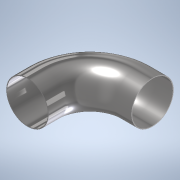
# Autodesk Inventor part: Kolano 90° ø101,6x2 R110
Saved by Autodesk Inventor 2020 (Build 240168000, 168)
## iProperties
RuleStatus: InUse
Created: 2021-10-14
Part Number: Kolano 90° ø101,6x2 R110
Material: 304L
Description: Kolano 90° ø101,6x2 R110
Document SubType Name: Modelowanie
Designer: inż. R.Jargiło
Density: 8 g/cm^3
Sheet Metal Rule: 1,5
Sheet Metal Width: 0,000 mm
Sheet Metal Length: 0,000 mm
Sheet Metal Area: 0,000 mm^2
Appearance: Częściowo polerowany(1)
Mass: 58.943 g
Surface Area: 91.7698 cm^2
Volume: 7.36788 cm^3
Project: 0479
Author: inż. R.Jargiło
Autodesk Inventor part; units mm, degrees
ref_plane "YZ Plane" through (0, 0, 0) normal (1, 0, 0) x (0, 1, 0)
ref_plane "XZ Plane" through (0, 0, 0) normal (0, 1, 0) x (-1, 0, 0)
sketch "Szkic6" plane through (0, 0, 0) normal (0, 0, 1) x (1, 0, 0)
  line L0 (-29.6067, 0) -> (35.2678, 0) construction
  line L1 (0, 42.3419) -> (0, -58.3726) construction
  arc A0 (110, 0) -> (0, -110) centre (110, -110) ccw
  line L2 (0, -110) -> (110, -110) construction
  line L3 (110, -110) -> (110, -44.4669) construction
  line L4 (110, 0) -> (150, 0)
  line L5 (0, -110) -> (0, -150)
  point P0 (0, 0)
  dimension "d24" = 110
  dimension "d31" = 90
  dimension "d36" = 40
  dimension "d37" = 40
  constraints: 8 end point, 4 point on line, 2 point on circle, 1 centre point, 1 horizontal, 1 tangent, 1 vertical alignment
  measures "d24" radius of A0
  measures "d31" angle of L2 L3
  measures "d36" distance of L4.start L4.end
  measures "d37" distance of L2.start L5.end
ref_plane "Płaszczyzna konstrukcyjna2" through (0, -110, 0) normal (0, -1, 0) x (1, 0, 0)
sketch "Szkic8" plane through (0, -110, 0) normal (0, -1, 0) x (1, 0, 0)
  circle A0 centre (0, 0) radius 50.8
  circle A1 centre (0, 0) radius 48.8
  dimension "d32" = 101.6
  dimension "d33" = 2
  constraints: 2 centre point, 1 coincident
  measures "d32" diameter of A0
  measures "d33" radial gap between concentric circles of A0 A1
sweep "Przeciągnięcie2" add profiles "Szkic8" path "Szkic6"
equation "\"d32\" = OD"
equation "\"d33\" = THK"
equation "\"d24\" = R"
equation "\"d31\" = KAT"
equation "\"d36\" = PROSTKA"
equation "\"d37\" = PROSTKA"
equation "\"SzerokośćGięciaPodcięcia\" = Grubość"
equation "\"RozmiarPodcięciaNarożnika\" = 4 * Grubość"
equation "\"PromieńPrzejścia\" = PromieńGięcia"
equation "\"Rozmiar_promienia_Jacobiego\" = PromieńGięcia"
equation "\"Wielk_odstępu\" = Grubość"
equation "\"d2\" = PromieńGięcia"
equation "\"d23\" = PromieńGięcia"
equation "\"R\" = 110"
equation "\"OD\" = 101.6"
equation "\"THK\" = 2"
equation "\"KAT\" = 90deg"
equation "\"PROSTKA\" = 40"
equation "\"Grubość\" = 1.5"
equation "\"PromieńGięcia\" = 3"
